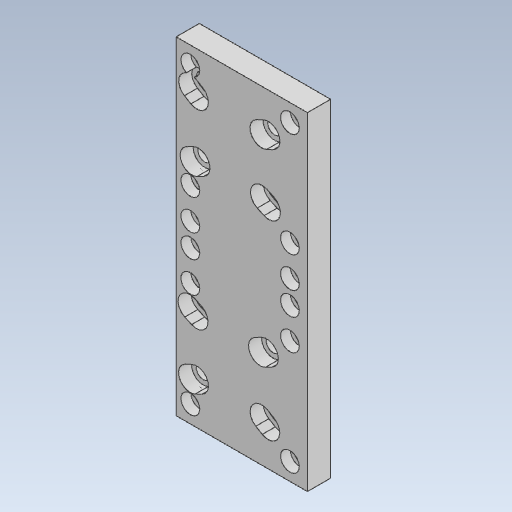
# Autodesk Inventor part: Z connection plate
Saved by Autodesk Inventor 2020 (Build 240168000, 168)
## iProperties
Created: 2019-05-25
Part Number: Z connection plate
Material: Generic
Document SubType Name: Modeling
Designer: LillaHunden
Density: 1 g/cm^3
Appearance: Default
Author: LillaHunden
Autodesk Inventor part; units mm, degrees
ref_plane "YZ Plane" through (0, 0, 0) normal (1, 0, 0) x (0, 1, 0)
ref_plane "XZ Plane" through (0, 0, 0) normal (0, 1, 0) x (-1, 0, 0)
ref_plane "XY Plane" through (0, 0, 0) normal (0, 0, 1) x (1, 0, 0)
sketch "Sketch1" plane through (0, 0, 0) normal (0, 0, 1) x (1, 0, 0)
  line L0 (-36.5524, -46.7459) -> (-66.2609, -46.7459) construction
  line L1 (-66.2609, -46.7459) -> (-66.2609, -56.6459) construction
  line L2 (-66.2609, -18.5459) -> (-36.5524, -18.5459) construction
  arc A0 (-30.8955, -24.2027) -> (-36.5524, -18.5459) centre (-33.7239, -21.3743) ccw construction
  line L3 (-30.8955, -24.2027) -> (-30.8955, -41.089) construction
  arc A1 (-36.5524, -46.7459) -> (-30.8955, -41.089) centre (-33.7239, -43.9175) ccw construction
  line L4 (-66.2609, 56.6459) -> (-20.9295, 56.6459)
  line L5 (-20.9295, 56.6459) -> (-20.9295, -56.6459)
  line L6 (-20.9295, -56.6459) -> (-66.2609, -56.6459)
  line L7 (-66.2609, -56.6459) -> (-66.2609, 56.6459)
  circle A2 centre (-26.9955, -4) radius 1.2295 projected
  circle A3 centre (-61.3755, 4) radius 1.2295 projected
  circle A4 centre (-26.9955, -50.6459) radius 1.2295 projected
  circle A5 centre (-61.3755, -14.6459) radius 1.2295 projected
  circle A6 centre (-26.9955, 14.6459) radius 1.2295 projected
  circle A7 centre (-26.9955, 50.6459) radius 1.2295 projected
  circle A8 centre (-61.3755, 50.6459) radius 1.2295 projected
  circle A9 centre (-61.3755, 14.6459) radius 1.2295 projected
  circle A10 centre (-26.9955, -14.6459) radius 1.2295 projected
  circle A11 centre (-61.3755, -50.6459) radius 1.2295 projected
  circle A12 centre (-26.9955, 4) radius 1.2295 projected
  circle A13 centre (-61.3755, -4) radius 1.2295 projected
  line L8 (-66.2609, 18.5459) -> (-66.2609, -18.5459) projected
  arc A14 (-30.8455, 41.089) -> (-36.5024, 46.7459) centre (-33.6739, 43.9175) ccw projected
  line L9 (-66.2609, 46.7459) -> (-36.5024, 46.7459) projected
  arc A15 (0.0303, -50.2581) -> (0.0303, -51.7044) centre (-3.9038, -50.9812) ccw projected
  arc A16 (0.0303, -34.2581) -> (0.0303, -35.7044) centre (-3.9038, -34.9812) ccw projected
  arc A17 (0.0303, 21.7419) -> (0.0303, 20.2956) centre (-3.9038, 21.0188) ccw projected
  arc A18 (0.0303, 47.4368) -> (0.0303, 45.9904) centre (-3.9038, 46.7136) ccw projected
  arc A19 (0.0303, -18.2581) -> (0.0303, -19.7044) centre (-3.9038, -18.9812) ccw projected
  line L10 (0.0303, -34.2581) -> (0.0303, -35.7044) projected
  line L11 (11.9038, -56.6459) -> (11.9038, -2.6124) projected
  line L12 (-4.1031, 56.6459) -> (-66.2609, 56.6459) projected
  line L13 (-66.2609, -56.6459) -> (11.9038, -56.6459) projected
  line L14 (0.0303, -50.2581) -> (0.0303, -51.7044) projected
  line L15 (0.0303, 21.7419) -> (0.0303, 20.2956) projected
  line L16 (0.0303, -18.2581) -> (0.0303, -19.7044) projected
  line L17 (0.0303, 47.4368) -> (0.0303, 45.9904) projected
  arc A20 (11.9038, -2.6124) -> (3.7292, 8.1531) centre (0.5689, -2.7331) ccw projected
  arc A21 (-0.8009, 14.5332) -> (3.7292, 8.1531) centre (5.4838, 14.1972) ccw projected
  arc A22 (-36.4527, 18.5459) -> (-30.8455, 24.252) centre (-33.6491, 21.3989) ccw projected
  line L18 (-36.4527, 18.5459) -> (-66.2609, 18.5459) projected
  arc A23 (2.7998, 20.6829) -> (3.7292, 22.3722) centre (1.7292, 22.3722) ccw projected
  line L19 (3.7292, 22.3722) -> (3.7292, 50.5278) projected
  arc A24 (3.7292, 50.5278) -> (3.1161, 52.6559) centre (-0.2708, 50.5278) ccw projected
  arc A25 (3.1161, 52.6559) -> (-4.1031, 56.6459) centre (-4.1031, 48.1199) ccw projected
  arc A26 (2.7998, 20.6829) -> (-0.8009, 14.5332) centre (6.9598, 14.1183) ccw projected
  line L20 (-66.2609, 56.6459) -> (-66.2609, 46.7459) projected
  line L21 (-30.8455, 41.089) -> (-30.8455, 24.252) projected
  point P0 (0, 0)
  point P1 (-1.9697, -56.6459)
  point P2 (11.9038, -23.2432)
  point P3 (11.9038, -14.7192)
  point P4 (0.0303, 56.6459)
  point P5 (-64.9755, 18.5459)
  point P6 (-66.2609, 18.5953)
  point P7 (-33.6739, 43.9175)
  point P8 (-33.6739, 43.9175)
  point P9 (-3.9038, 21.0188)
  point P10 (-33.6739, 43.9175)
  point P11 (-3.9038, -18.9812)
  point P12 (-33.6739, 43.9175)
  point P13 (-33.6491, 21.3989)
  point P14 (-33.6739, 43.9175)
  point P15 (-33.6491, 21.3989)
  point P16 (-33.6739, 43.9175)
  point P17 (-33.6491, 21.3989)
  point P18 (-33.6739, 43.9175)
  point P19 (-33.6491, 21.3989)
  point P20 (-33.6739, 43.9175)
  point P21 (-33.6491, 21.3989)
  constraints: 8 end point, 2 parallel, 1 horizontal, 1 perpendicular
extrude "Extrusion1" add sketch "Sketch1" along normal blind 8 contours L4 L5 L6 L7 L18 A22 L21 A14 L9 | L9 A14 L21 A22 L18 L7 | A2 | A3 | A4 | A5 | A6 | A7 | A8 | A9 | A10 | A11 | A12 | A13
sketch "Sketch2" plane through (0, 0, 8) normal (0, 0, 1) x (1, 0, 0)
  circle A0 centre (-34.2455, 22.0059) radius 1.621 construction
  circle A1 centre (-61.3755, 43.9159) radius 1.621 construction
  circle A2 centre (-60.8955, 22.0259) radius 1.621 construction
  circle A3 centre (-34.4255, 43.2959) radius 1.621 construction
  line L0 (-30.9455, 18.6459) -> (-64.8755, 18.6459) construction
  line L1 (-30.9455, 46.6459) -> (-30.9455, 18.6459) construction
  line L2 (-64.8755, 46.6459) -> (-30.9455, 46.6459) construction
  line L3 (-64.8755, 18.6459) -> (-64.8755, 46.6459) construction
  circle A4 centre (-61.6255, -22.0059) radius 1.621 construction
  circle A5 centre (-34.4955, -43.9159) radius 1.621 construction
  circle A6 centre (-34.9755, -22.0259) radius 1.621 construction
  circle A7 centre (-61.4455, -43.2959) radius 1.621 construction
  line L4 (-64.9255, -18.6459) -> (-30.9955, -18.6459) construction
  line L5 (-64.9255, -46.6459) -> (-64.9255, -18.6459) construction
  line L6 (-30.9955, -46.6459) -> (-64.9255, -46.6459) construction
  line L7 (-30.9955, -18.6459) -> (-30.9955, -46.6459) construction
  line L8 (-61.3755, 50.6459) -> (-26.9955, 50.6459) construction
  line L9 (-26.9955, 50.6459) -> (-26.9955, 14.6459) construction
  line L10 (-26.9955, 14.6459) -> (-61.3755, 14.6459) construction
  line L11 (-61.3755, 14.6459) -> (-61.3755, 50.6459) construction
  line L12 (-61.3755, -14.6459) -> (-26.9955, -14.6459) construction
  line L13 (-26.9955, -14.6459) -> (-26.9955, -50.6459) construction
  line L14 (-26.9955, -50.6459) -> (-61.3755, -50.6459) construction
  line L15 (-61.3755, -50.6459) -> (-61.3755, -14.6459) construction
  line L16 (-61.3755, 14.6459) -> (-26.9955, 14.6459) construction
  line L17 (-26.9955, 14.6459) -> (-26.9955, 4) construction
  line L18 (-26.9955, 4) -> (-61.3755, 4) construction
  line L19 (-61.3755, 4) -> (-61.3755, 14.6459) construction
  line L20 (-61.3755, -14.6459) -> (-26.9955, -14.6459) construction
  line L21 (-26.9955, -14.6459) -> (-26.9955, -4) construction
  line L22 (-26.9955, -4) -> (-61.3755, -4) construction
  line L23 (-61.3755, -4) -> (-61.3755, -14.6459) construction
  line L24 (-29.2136, 14.6459) -> (-29.2136, -14.6459) construction
  line L25 (-29.2136, 0) -> (-59.8245, 0) construction
  line L26 (-66.2609, 56.6459) -> (-66.2609, -56.6459) projected
  point P0 (0, 0)
  dimension "d2" = 4
  dimension "d3" = 4
  dimension "d4" = 4
  dimension "d5" = 4
  dimension "d6" = 4
  dimension "d7" = 4
  dimension "d8" = 4
  constraints: 36 end point, 12 coincident, 8 parallel, 5 horizontal, 5 perpendicular, 4 point on line, 1 midpoint, 1 vertical alignment
  measures "d2" distance between parallel lines of L4 L12
  measures "d3" distance between parallel lines of L14 L6
  measures "d4" distance between parallel lines of L7 L13
  measures "d5" distance between parallel lines of L10 L0
  measures "d6" distance between parallel lines of L2 L8
  measures "d7" distance between parallel lines of L25 L22
  measures "d8" distance between parallel lines of L25 L18
sketch "Sketch3" plane through (0, 0, 8) normal (0, 0, 1) x (1, 0, 0)
  point P0 (-26.9955, 50.6459)
  point P1 (-61.3755, 50.6459)
  point P2 (-26.9955, 14.6459)
  point P3 (-61.3755, 14.6459)
  point P4 (-61.3755, -14.6459)
  point P5 (-26.9955, -14.6459)
  point P6 (-26.9955, -50.6459)
  point P7 (-61.3755, -50.6459)
  point P8 (-61.3755, 4)
  point P9 (-26.9955, 4)
  point P10 (-26.9955, -4)
  point P11 (-61.3755, -4)
hole "Hole1" at (-26.9955, 50.6459, 8) at (-61.3755, 50.6459, 8) at (-26.9955, 14.6459, 8) at (-61.3755, 14.6459, 8) at (-61.3755, -14.6459, 8) at (-26.9955, -14.6459, 8) at (-26.9955, -50.6459, 8) at (-61.3755, -50.6459, 8) at (-61.3755, 4, 8) at (-26.9955, 4, 8) at (-26.9955, -4, 8) at (-61.3755, -4, 8) direction (0, 0, -1) diameter 3.6 depth 8 counterbore diameter 6.5 counterbore depth 3.4
sketch "Sketch4" plane through (0, 0, 8) normal (0, 0, 1) x (1, 0, 0)
  point P0 (-34.4255, 43.2959)
  point P1 (-61.3755, 43.9159)
  point P2 (-60.8955, 22.0259)
  point P3 (-34.2455, 22.0059)
hole "Hole3" at (-34.4255, 43.2959, 8) at (-61.3755, 43.9159, 8) at (-60.8955, 22.0259, 8) at (-34.2455, 22.0059, 8) direction (0, 0, -1) diameter 4.8 depth 8 counterbore diameter 8 counterbore depth 4.5
sketch "Sketch5" plane through (0, 0, 8) normal (0, 0, 1) x (1, 0, 0)
  point P0 (-61.6255, -22.0059)
  point P1 (-34.4955, -43.9159)
  point P2 (-34.9755, -22.0259)
  point P3 (-61.4455, -43.2959)
hole "Hole5" at (-61.6255, -22.0059, 8) at (-34.4955, -43.9159, 8) at (-34.9755, -22.0259, 8) at (-61.4455, -43.2959, 8) direction (0, 0, -1) diameter 4.8 depth 8 counterbore diameter 8 counterbore depth 4.5
sketch "Sketch6" plane through (0, 0, 0) normal (0, 0, -1) x (-1, 0, 0)
  circle A0 centre (61.6255, -22.0059) radius 1.621 construction
  circle A1 centre (34.4955, -43.9159) radius 1.621 construction
  circle A2 centre (34.9755, -22.0259) radius 1.621 construction
  circle A3 centre (61.4455, -43.2959) radius 1.621 construction
  line L0 (64.9255, -18.6459) -> (30.9955, -18.6459) construction
  line L1 (64.9255, -46.6459) -> (64.9255, -18.6459) construction
  line L2 (30.9955, -46.6459) -> (64.9255, -46.6459) construction
  line L3 (30.9955, -18.6459) -> (30.9955, -46.6459) construction
  circle A4 centre (34.2455, 22.0059) radius 1.621 construction
  circle A5 centre (61.3755, 43.9159) radius 1.621 construction
  circle A6 centre (60.8955, 22.0259) radius 1.621 construction
  circle A7 centre (34.4255, 43.2959) radius 1.621 construction
  line L4 (30.9455, 18.6459) -> (64.8755, 18.6459) construction
  line L5 (30.9455, 46.6459) -> (30.9455, 18.6459) construction
  line L6 (64.8755, 46.6459) -> (30.9455, 46.6459) construction
  line L7 (64.8755, 18.6459) -> (64.8755, 46.6459) construction
  line L8 (32.9455, 36.6459) -> (62.8755, 36.6459)
  line L9 (62.8755, 36.6459) -> (62.8755, 28.6459)
  line L10 (62.8755, 28.6459) -> (32.9455, 28.6459)
  line L11 (32.9455, 28.6459) -> (32.9455, 36.6459)
  line L12 (43.9105, 44.6459) -> (51.9105, 44.6459)
  line L13 (51.9105, 44.6459) -> (51.9105, 20.6459)
  line L14 (51.9105, 20.6459) -> (43.9105, 20.6459)
  line L15 (43.9105, 20.6459) -> (43.9105, 44.6459)
  line L16 (43.9605, -20.6459) -> (51.9605, -20.6459)
  line L17 (51.9605, -20.6459) -> (51.9605, -44.6459)
  line L18 (51.9605, -44.6459) -> (43.9605, -44.6459)
  line L19 (43.9605, -44.6459) -> (43.9605, -20.6459)
  line L20 (32.9955, -28.6459) -> (62.9255, -28.6459)
  line L21 (62.9255, -28.6459) -> (62.9255, -36.6459)
  line L22 (62.9255, -36.6459) -> (32.9955, -36.6459)
  line L23 (32.9955, -36.6459) -> (32.9955, -28.6459)
  point P0 (0, 0)
  point P1 (47.9105, 44.6459)
  point P2 (47.9105, 46.6459)
  point P3 (32.9455, 32.6459)
  point P4 (30.9455, 32.6459)
  point P5 (47.9605, -20.6459)
  point P6 (47.9605, -18.6459)
  point P7 (62.9255, -32.6459)
  point P8 (64.9255, -32.6459)
  point P9 (51.9105, 28.6459)
  point P10 (51.9105, 36.6459)
  point P11 (43.9105, 36.6459)
  point P12 (43.9105, 28.6459)
  point P13 (43.9605, -36.6459)
  point P14 (51.9605, -36.6459)
  point P15 (51.9605, -28.6459)
  point P16 (43.9605, -28.6459)
  dimension "d31" = 2
  dimension "d32" = 2
  dimension "d33" = 2
  dimension "d34" = 2
  dimension "d35" = 8
  dimension "d36" = 8
  dimension "d37" = 8
  dimension "d38" = 8
  dimension "d39" = 2
  dimension "d40" = 2
  dimension "d41" = 2
  dimension "d42" = 2
  constraints: 32 end point, 8 midpoint, 8 parallel, 4 horizontal, 4 perpendicular, 2 horizontal alignment, 2 vertical alignment
  measures "d31" distance between parallel lines of L4 L14
  measures "d32" distance between parallel lines of L6 L12
  measures "d33" distance between parallel lines of L5 L11
  measures "d34" distance between parallel lines of L7 L9
  measures "d35" distance of L13.end L14.end
  measures "d36" distance of L10.end L8.start
  measures "d37" distance of L22.end L20.start
  measures "d38" distance of L17.end L18.end
  measures "d39" distance between parallel lines of L2 L18
  measures "d40" distance between parallel lines of L0 L16
  measures "d41" distance between parallel lines of L3 L23
  measures "d42" distance between parallel lines of L1 L21
extrude "Extrusion2" add sketch "Sketch6" along normal blind 1.8
fillet "Fillet1" radius 4.1 8 edges at (-51.9605, -36.6459, -0.9) (-43.9605, -36.6459, -0.9) (-43.9605, -28.6459, -0.9) (-51.9605, -28.6459, -0.9) (-43.9105, 28.6459, -0.9) (-51.9105, 28.6459, -0.9) (-51.9105, 36.6459, -0.9) (-43.9105, 36.6459, -0.9)
sketch "Sketch7" plane through (0, 0, 8) normal (0, 0, 1) x (1, 0, 0)
  arc A0 (-56.0105, 36.6459) -> (-51.9105, 40.7459) centre (-56.0105, 40.7459) ccw projected
  arc A1 (-51.9105, 24.5459) -> (-56.0105, 28.6459) centre (-56.0105, 24.5459) ccw projected
  arc A2 (-39.8105, 28.6459) -> (-43.9105, 24.5459) centre (-39.8105, 24.5459) ccw projected
  arc A3 (-43.9105, 40.7459) -> (-39.8105, 36.6459) centre (-39.8105, 40.7459) ccw projected
  arc A4 (-51.9605, -40.7459) -> (-56.0605, -36.6459) centre (-56.0605, -40.7459) ccw projected
  arc A5 (-39.8605, -36.6459) -> (-43.9605, -40.7459) centre (-39.8605, -40.7459) ccw projected
  arc A6 (-43.9605, -24.5459) -> (-39.8605, -28.6459) centre (-39.8605, -24.5459) ccw projected
  arc A7 (-56.0605, -28.6459) -> (-51.9605, -24.5459) centre (-56.0605, -24.5459) ccw projected
  arc A8 (-62.7152, 47.6849) -> (-60.0358, 47.6849) centre (-61.3755, 43.9159) ccw projected
  line L0 (-61.3755, 43.9159) -> (-56.0105, 40.7459) construction
  line L1 (-61.3755, 43.9159) -> (-59.1371, 42.5933) construction
  line L2 (-63.4103, 40.4721) -> (-61.1719, 39.1495)
  line L3 (-57.1023, 46.037) -> (-59.3407, 47.3596)
  arc A9 (-59.3407, 47.3596) -> (-63.4103, 40.4721) centre (-61.3755, 43.9159) ccw
  arc A10 (-61.1719, 39.1495) -> (-57.1023, 46.037) centre (-59.1371, 42.5933) ccw
  circle A11 centre (-34.4255, 43.2959) radius 2.4 projected
  line L4 (-34.4255, 43.2959) -> (-39.8105, 40.7459) construction
  circle A12 centre (-34.2455, 22.0059) radius 2.4 construction
  line L5 (-34.2455, 22.0059) -> (-39.8105, 24.5459) construction
  circle A13 centre (-61.6255, -22.0059) radius 2.4 construction
  line L6 (-61.6255, -22.0059) -> (-56.0605, -24.5459) construction
  circle A14 centre (-34.9755, -22.0259) radius 2.4 construction
  line L7 (-39.8605, -24.5459) -> (-34.9755, -22.0259) construction
  circle A15 centre (-61.4455, -43.2959) radius 2.4 construction
  line L8 (-61.4455, -43.2959) -> (-56.0605, -40.7459) construction
  circle A16 centre (-34.4955, -43.9159) radius 2.4 construction
  line L9 (-34.4955, -43.9159) -> (-39.8605, -40.7459) construction
  line L10 (-34.4255, 43.2959) -> (-36.7754, 42.1831) construction
  line L11 (-36.1374, 46.911) -> (-38.4873, 45.7983)
  line L12 (-35.0635, 38.568) -> (-32.7136, 39.6807)
  arc A17 (-32.7136, 39.6807) -> (-36.1374, 46.911) centre (-34.4255, 43.2959) ccw
  arc A18 (-38.4873, 45.7983) -> (-35.0635, 38.568) centre (-36.7754, 42.1831) ccw
  line L13 (-34.2455, 22.0059) -> (-36.6108, 23.0854) construction
  line L14 (-32.5846, 25.6448) -> (-34.9499, 26.7243)
  line L15 (-38.2717, 19.4466) -> (-35.9064, 18.367)
  arc A19 (-35.9064, 18.367) -> (-32.5846, 25.6448) centre (-34.2455, 22.0059) ccw
  arc A20 (-34.9499, 26.7243) -> (-38.2717, 19.4466) centre (-36.6108, 23.0854) ccw
  line L16 (-61.6255, -22.0059) -> (-59.2602, -23.0854) construction
  line L17 (-59.9646, -18.367) -> (-57.5994, -19.4466)
  line L18 (-60.9211, -26.7243) -> (-63.2864, -25.6448)
  arc A21 (-59.9646, -18.367) -> (-63.2864, -25.6448) centre (-61.6255, -22.0059) ccw
  arc A22 (-60.9211, -26.7243) -> (-57.5994, -19.4466) centre (-59.2602, -23.0854) ccw
  line L19 (-34.9755, -22.0259) -> (-37.2862, -23.2179) construction
  line L20 (-36.8093, -18.471) -> (-39.12, -19.663)
  line L21 (-35.4524, -26.7727) -> (-33.1417, -25.5807)
  arc A23 (-33.1417, -25.5807) -> (-36.8093, -18.471) centre (-34.9755, -22.0259) ccw
  arc A24 (-39.12, -19.663) -> (-35.4524, -26.7727) centre (-37.2862, -23.2179) ccw
  line L22 (-61.4455, -43.2959) -> (-59.0957, -42.1831) construction
  line L23 (-59.7336, -46.911) -> (-57.3838, -45.7983)
  line L24 (-60.8076, -38.568) -> (-63.1574, -39.6807)
  arc A25 (-63.1574, -39.6807) -> (-59.7336, -46.911) centre (-61.4455, -43.2959) ccw
  arc A26 (-57.3838, -45.7983) -> (-60.8076, -38.568) centre (-59.0957, -42.1831) ccw
  line L25 (-34.4955, -43.9159) -> (-36.734, -42.5933) construction
  line L26 (-32.4607, -40.4721) -> (-34.6992, -39.1495)
  line L27 (-38.7688, -46.037) -> (-36.5303, -47.3596)
  arc A27 (-36.5303, -47.3596) -> (-32.4607, -40.4721) centre (-34.4955, -43.9159) ccw
  arc A28 (-34.6992, -39.1495) -> (-38.7688, -46.037) centre (-36.734, -42.5933) ccw
  circle A29 centre (-34.4255, 43.2959) radius 4 projected
  circle A30 centre (-34.2455, 22.0059) radius 4 projected
  circle A31 centre (-61.6255, -22.0059) radius 4 projected
  circle A32 centre (-34.9755, -22.0259) radius 4 projected
  circle A33 centre (-34.4955, -43.9159) radius 4 projected
  circle A34 centre (-61.4455, -43.2959) radius 4 projected
  circle A35 centre (-60.8955, 22.0259) radius 2.4 projected
  line L28 (-60.8955, 22.0259) -> (-56.0105, 24.5459) construction
  line L29 (-60.8955, 22.0259) -> (-58.5849, 23.2179) construction
  line L30 (-62.7293, 25.5807) -> (-60.4187, 26.7727)
  line L31 (-56.751, 19.663) -> (-59.0617, 18.471)
  arc A36 (-62.7293, 25.5807) -> (-59.0617, 18.471) centre (-60.8955, 22.0259) ccw
  arc A37 (-56.751, 19.663) -> (-60.4187, 26.7727) centre (-58.5849, 23.2179) ccw
  circle A38 centre (-60.8955, 22.0259) radius 4 projected
  point P0 (0, 0)
  point P1 (-60.2563, 43.2546)
  point P2 (-58.693, 42.3309)
  point P3 (-35.6004, 42.7395)
  point P4 (-35.4282, 22.5457)
  point P5 (-60.4429, -22.5457)
  point P6 (-36.1309, -22.6219)
  point P7 (-60.2706, -42.7395)
  point P8 (-35.6147, -43.2546)
  point P9 (-37.028, 23.2759)
  point P10 (-58.843, -23.2759)
  point P11 (-37.418, -23.2859)
  point P12 (-37.178, -42.3309)
  point P13 (-58.753, -42.0209)
  point P14 (-59.7402, 22.6219)
  point P15 (-58.453, 23.2859)
  point P16 (-60.0358, 47.6849)
  dimension "d46" = 2.6
  dimension "d47" = 2.6
  dimension "d48" = 2.6
  dimension "d49" = 2.6
  dimension "d50" = 2.6
  dimension "d51" = 2.6
  dimension "d52" = 2.6
  dimension "d53" = 2.6
  constraints: 80 end point, 40 tangent, 32 point on circle, 16 centre point, 15 midpoint, 8 parallel, 8 point on line, 1 concentric
  measures "d46" distance of L2.start L2.end
  measures "d47" distance of L30.start L30.end
  measures "d48" distance of L11.start L11.end
  measures "d49" distance of L14.start L14.end
  measures "d50" distance of L17.start L17.end
  measures "d51" distance of L20.start L20.end
  measures "d52" distance of L24.start L24.end
  measures "d53" distance of L26.start L26.end
extrude "Extrusion3" cut sketch "Sketch7" against normal up to surface (4.5 mm away) contours A9 A8 | A8 L3 A10 L2 | A11 | A29 L12 A18 L11 | A17 A29 | A30 L15 A20 L14 | A19 A30 | A31 A21 | L17 A22 L18 A31 | A32 L21 A24 L20 | A34 L24 A26 L23 | A25 A34 | A33 L27 A28 L26 | A27 A33 | A35 | A38 A36 | L30 A37 L31 A38
sketch "Sketch8" plane through (-61.3755, 43.9159, 3.5) normal (0, 0, 1) x (0.8609425, -0.5087023, 0)
  line L0 (0, 0) -> (2.6, 0) construction
  line L1 (0, -2.4) -> (2.6, -2.4)
  line L2 (2.6, 2.4) -> (0, 2.4)
  arc A0 (0, 2.4) -> (0, -2.4) centre (0, 0) ccw
  arc A1 (2.6, -2.4) -> (2.6, 2.4) centre (2.6, 0) ccw
  circle A2 centre (0, 0) radius 2.4 projected
  line L3 (0, 0) -> (6.2315, 0) construction
  arc A3 (2.6, -4) -> (2.6, 4) centre (2.6, 0) ccw construction
  line L4 (23.5178, 13.1757) -> (22.0608, 11.0224) construction
  line L5 (21.5301, 14.5207) -> (20.073, 12.3673)
  line L6 (24.0485, 9.6774) -> (25.5055, 11.8308)
  arc A4 (25.5055, 11.8308) -> (21.5301, 14.5207) centre (23.5178, 13.1757) ccw
  arc A5 (20.073, 12.3673) -> (24.0485, 9.6774) centre (22.0608, 11.0224) ccw
  line L7 (23.5178, 13.1757) -> (20.1788, 8.241) construction
  circle A6 centre (23.5178, 13.1757) radius 2.4 projected
  arc A7 (18.7479, 13.2639) -> (25.3737, 8.7808) centre (22.0608, 11.0224) ccw construction
  line L8 (11.5487, -18.6019) -> (12.9317, -16.4002) construction
  line L9 (34.503, -5.0622) -> (31.9175, -5.3359) construction
  line L10 (33.3193, -56.882) -> (39.4026, -56.2379) construction
  line L11 (44.3046, -75.1199) -> (47.6435, -70.1852) construction
  line L12 (56.2736, -43.3423) -> (54.8906, -45.544) construction
  circle A8 centre (11.5487, -18.6019) radius 2.4 projected
  line L13 (11.5487, -18.6019) -> (12.9317, -16.4002) construction
  line L14 (13.5811, -19.8785) -> (14.964, -17.6768)
  line L15 (10.8994, -15.1236) -> (9.5164, -17.3253)
  arc A9 (9.5164, -17.3253) -> (13.5811, -19.8785) centre (11.5487, -18.6019) ccw
  arc A10 (14.964, -17.6768) -> (10.8994, -15.1236) centre (12.9317, -16.4002) ccw
  line L16 (34.503, -5.0622) -> (31.9175, -5.3359) construction
  line L17 (34.2503, -2.6755) -> (31.6648, -2.9493)
  line L18 (32.1702, -7.7226) -> (34.7558, -7.4488)
  arc A11 (34.7558, -7.4488) -> (34.2503, -2.6755) centre (34.503, -5.0622) ccw
  arc A12 (31.6648, -2.9493) -> (32.1702, -7.7226) centre (31.9175, -5.3359) ccw
  line L19 (33.3193, -56.882) -> (35.9049, -56.6082) construction
  line L20 (33.572, -59.2687) -> (36.1576, -58.9949)
  line L21 (35.6521, -54.2216) -> (33.0666, -54.4954)
  arc A13 (33.0666, -54.4954) -> (33.572, -59.2687) centre (33.3193, -56.882) ccw
  arc A14 (36.1576, -58.9949) -> (35.6521, -54.2216) centre (35.9049, -56.6082) ccw
  line L22 (56.2736, -43.3423) -> (54.8906, -45.544) construction
  line L23 (54.2413, -42.0657) -> (52.8583, -44.2674)
  line L24 (56.9229, -46.8206) -> (58.3059, -44.6189)
  arc A15 (58.3059, -44.6189) -> (54.2413, -42.0657) centre (56.2736, -43.3423) ccw
  arc A16 (52.8583, -44.2674) -> (56.9229, -46.8206) centre (54.8906, -45.544) ccw
  line L25 (44.3046, -75.1199) -> (45.7616, -72.9665) construction
  line L26 (42.3168, -73.775) -> (43.7738, -71.6216)
  line L27 (47.7493, -74.3115) -> (46.2923, -76.4649)
  arc A17 (42.3168, -73.775) -> (46.2923, -76.4649) centre (44.3046, -75.1199) ccw
  arc A18 (47.7493, -74.3115) -> (43.7738, -71.6216) centre (45.7616, -72.9665) ccw
  circle A19 centre (44.3046, -75.1199) radius 2.4 projected
  circle A20 centre (33.3193, -56.882) radius 2.4 projected
  circle A21 centre (56.2736, -43.3423) radius 2.4 projected
  arc A22 (51.5034, -43.4163) -> (58.2778, -47.6717) centre (54.8906, -45.544) ccw projected
  arc A23 (36.3261, -60.586) -> (35.4837, -52.6305) centre (35.9049, -56.6082) ccw projected
  line L28 (67.8223, -61.9442) -> (65.2223, -61.9442) construction
  line L29 (67.8223, -59.5442) -> (65.2223, -59.5442)
  line L30 (65.2223, -64.3442) -> (67.8223, -64.3442)
  arc A24 (67.8223, -64.3442) -> (67.8223, -59.5442) centre (67.8223, -61.9442) ccw
  arc A25 (65.2223, -59.5442) -> (65.2223, -64.3442) centre (65.2223, -61.9442) ccw
  arc A26 (67.8223, -65.9442) -> (67.8223, -57.9442) centre (67.8223, -61.9442) ccw projected
  arc A27 (65.2223, -57.9442) -> (65.2223, -65.9442) centre (65.2223, -61.9442) ccw projected
  arc A28 (49.0745, -75.2081) -> (42.4487, -70.7249) centre (45.7616, -72.9665) ccw projected
  arc A29 (40.9917, -72.8783) -> (47.6175, -77.3615) centre (44.3046, -75.1199) ccw projected
  arc A30 (31.4963, -1.3582) -> (32.3387, -9.3137) centre (31.9175, -5.3359) ccw projected
  arc A31 (16.3189, -18.5278) -> (9.5445, -14.2725) centre (12.9317, -16.4002) ccw projected
  circle A32 centre (34.503, -5.0622) radius 2.4 projected
  circle A33 centre (67.8223, -61.9442) radius 2.4 projected
  point P0 (75.1809, -6.5872)
  point P1 (1.3, 0)
  point P2 (22.7893, 12.0991)
  point P3 (21.8483, 10.7084)
  point P4 (12.2402, -17.501)
  point P5 (33.2103, -5.199)
  point P6 (34.6121, -56.7451)
  point P7 (55.5821, -44.4432)
  point P8 (45.0331, -74.0432)
  point P9 (66.5223, -61.9442)
  point P10 (67.8223, -64.3442)
  point P11 (67.8223, -59.5442)
  point P12 (33.0666, -54.4954)
  point P13 (33.572, -59.2687)
  point P14 (54.2413, -42.0657)
  point P15 (34.7558, -7.4488)
  point P16 (34.2503, -2.6755)
  point P17 (9.5164, -17.3253)
  point P18 (13.5811, -19.8785)
  point P19 (25.5055, 11.8308)
  point P20 (21.5301, 14.5207)
  point P21 (0, 2.4)
  point P22 (0, -2.4)
  constraints: 64 end point, 40 tangent, 32 point on circle, 16 centre point, 15 concentric, 9 midpoint, 8 parallel, 2 point on line, 1 horizontal
extrude "Extrusion4" cut sketch "Sketch8" against normal through all contours A2 L2 A1 L1 | A6 L6 A5 L5 | A8 L15 A10 L14 | A32 L18 A12 L17 | A20 L21 A14 L20 | A21 L24 A16 L23 | L26 A18 L27 A19 | A33 L30 A25 L29
equation "\"d8\" = d7"
equation "\"d36\" = d35"
equation "\"d37\" = d35"
equation "\"d38\" = d37"
equation "\"d39\" = d31"
equation "\"d40\" = d32"
equation "\"d41\" = d33"
equation "\"d42\" = d34"
equation "\"d47\" = d46"
equation "\"d48\" = d46"
equation "\"d49\" = d48"
equation "\"d50\" = d47"
equation "\"d51\" = d50"
equation "\"d52\" = d50"
equation "\"d53\" = d51"
body "Solid1"
